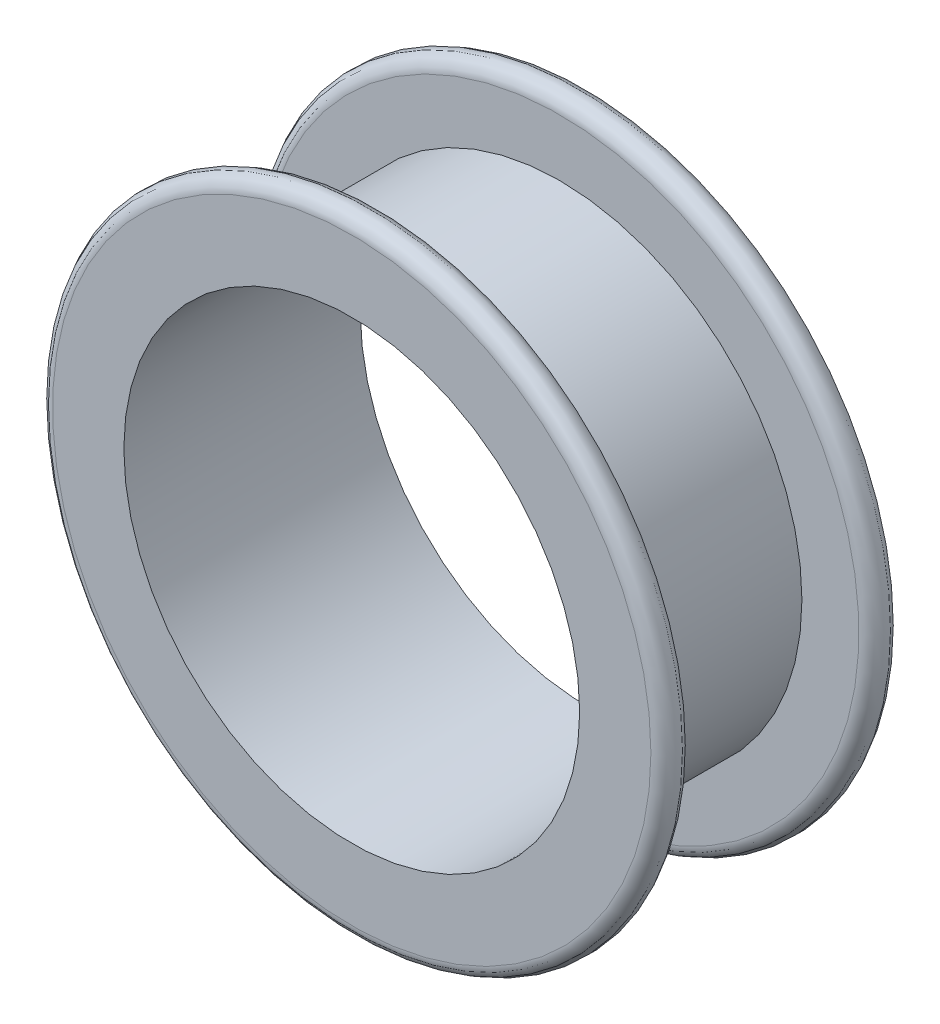
# Autodesk Inventor part: Prusa_pulley_thin
Saved by Autodesk Inventor 2019.3 (Build 233278000, 278)
## iProperties
Created: 2020-09-10
Part Number: Prusa_pulley_thin
Material: Generisch
Document SubType Name: Modeling
Designer: Nicolas Frick
Density: 1 g/cm^3
Appearance: Vorgabe
Author: Nicolas Frick
Autodesk Inventor part; units mm, degrees
ref_plane "YZ Plane" through (0, 0, 0) normal (1, 0, 0) x (0, 1, 0)
ref_plane "XZ Plane" through (0, 0, 0) normal (0, 1, 0) x (-1, 0, 0)
ref_plane "XY Plane" through (0, 0, 0) normal (0, 0, 1) x (1, 0, 0)
ref_plane "Arbeitsebene1" through (-327.6157, -655.2314, -332.6157) normal (0, 0, -1) x (-1, 0, 0)
sketch "Skizze1" plane through (-327.6157, -655.2314, -332.6157) normal (0, 0, -1) x (-1, 0, 0)
  circle A0 centre (-319.6057, 655.2314) radius 8 projected
  circle A1 centre (-319.6057, 655.2314) radius 8.5
  point P0 (-327.6157, 655.2314)
  dimension "d0" = 17
  constraints: 1 centre point, 1 coincident
  measures "d0" diameter of A1
extrude "Extrusion1" add sketch "Skizze1" along normal blind 6.3
sketch "Skizze2" plane through (-8.01, 0, -338.9157) normal (0, 0, -1) x (-1, 0, 0)
  circle A0 centre (0, 0) radius 11
  circle A1 centre (0, 0) radius 8
  point P0 (-8.01, 0)
  constraints: 2 centre point, 1 coincident
extrude "Extrusion3" add sketch "Skizze2" along normal blind 1
sketch "Skizze3" plane through (-8.01, 0, -332.6157) normal (0, 0, 1) x (1, 0, 0)
  circle A0 centre (0, 0) radius 8
  circle A1 centre (0, 0) radius 11
  point P0 (8.01, 0)
  constraints: 2 centre point, 1 coincident
extrude "Extrusion4" add sketch "Skizze3" along normal blind 1
fillet "Rundung1" radius 0.5 2 edges at (-19.01, 0, -331.6157) (2.99, 0, -339.9157)
fillet "Rundung2" radius 0.5 2 edges at (2.99, 0, -338.9157) (-19.01, 0, -332.6157)
